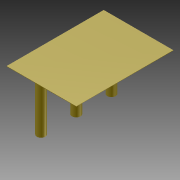
# Autodesk Inventor part: B12APtrmnls
Saved by Autodesk Inventor 2011 SP1 (Build 150282100, 282)
## iProperties
Created: 2013-12-24
Part Number: B12APtrmnls
Catalog Web Link: www.cadenas.de
Description: B Series - Terminals-
Vendor: NKKSWITCHES
Document SubType Name: Modeling
Designer: PARTuser1
Manufacturer: NKKSWITCHES
Density: 1 g/cm^3
Category: PARTsolutions
Company: NKKSWITCHES
Title: B12APtrmnls
Author: Cadenas PARTsolutions
PSOL_IDENT_0: {$CADENAS_DATA\23d-libs\nkkswitches\toggle\b\parts\b_terminals.prj},209 {VTYP=3D},{NB=B12APtrmnls},{
PSOL_IDENT_1: LINA=B12APtrmnls},{NN=B Series - Terminals},{DATE=06.03.2009 07:37:56},{GEOMDATE=28.01.2009 09:08:00
PSOL_IDENT_2: },{VERSION=},{LINEID=10},{LINESUBID=-1},{WBVAR=PLS,CRCTS,TGGLS,TRMNLS,CPS,CCLR}  {NB=B12APtrmnls},{L
PSOL_IDENT_3: INA=B12APtrmnls},{KT=DUMMY},{PN=B12AP},{SRS=B},{PLS=1},{CRCTS=2},{CRCTSALG= '2','2 - ON/NONE/ON','3'
PSOL_IDENT_4: ,'3 - ON/OFF/ON','5','5 - ON/NONE/(ON)','R','R - (ON)/NONE/ON','8','8 - (ON)/OFF/(ON)','9','9 - ON/O
PSOL_IDENT_5: FF/(ON)','S','S - (ON)/OFF/ON' },{TGGLS=A},{TGGLSALG=  'A','A - .394\" (10.0 mm) Bat','A1','A1 - .31
PSOL_IDENT_6: 5\" (8.0 mm) Bat with Panel Seal Threaded Bushing  '  ,'J','J - .248\" (6.3 mm) Bat','E','E - .394\"
PSOL_IDENT_7: (10.0 mm) Flatted','H','H - .248\" (6.3 mm) Flatted','K','K - Snap Top for Paddles','L','L - Lockin
PSOL_IDENT_8: g Lever' },{TRMNLS=P},{TRMNLSALG= 'P','P - Straight','B','B - Straight with Bracket', 'H','H - Right
PSOL_IDENT_9: Angle with Bracket','V','V - Vertical with Bracket' ,'W','W - Straight Long' },{CPS=},{CPSALG= '','
PSOL_IDENT_10: w/o Cap','G','G - .394\" (10.0 mm) Bat Lever Cap' },{CCLR=},{CCLR1= '', 'N/A' }
CNS_NN: B Series - Terminals
CNS_NB: B12APtrmnls
CNS_NBSYN: $PN.trmnls
CNS_LINA: B12APtrmnls
CNS_PN: B12AP
CNS_SRS: B
CNS_PLS: 1 - SPDT
CNS_CRCTS: 2 - ON/NONE/ON
CNS_CRCTSALG: '2','2 - ON/NONE/ON','3','3 - ON/OFF/ON','5','5 - ON/NONE/(ON)','R','R - (ON)/NONE/ON','8','8 - (ON)/OFF/(ON)','9','9 - ON/OFF/(ON)','S','S - (ON)/OFF/ON'
CNS_TGGLS: A - .394" (10.0 mm) Bat
CNS_TGGLSALG: 'A','A - .394" (10.0 mm) Bat','A1','A1 - .315" (8.0 mm) Bat with Panel Seal Threaded Bushing  '  ,'J','J - .248" (6.3 mm) Bat','E','E - .394" (10.0 mm) Flatted','H','H - .248" (6.3 mm) Flatted','K','K - Snap Top for Paddles','L','L - Locking Lever'
CNS_TRMNLS: P - Straight
CNS_TRMNLSALG: 'P','P - Straight','B','B - Straight with Bracket', 'H','H - Right Angle with Bracket','V','V - Vertical with Bracket' ,'W','W - Straight Long'
CNS_CPS: w/o Cap
CNS_CPSALG: '','w/o Cap','G','G - .394" (10.0 mm) Bat Lever Cap'
CNS_CCLR: N/A
CNS_CCLR1: '', 'N/A'
SUPPLIER: NKKSWITCHES
ARTICLENO: B12APtrmnls
BOMINFO: B12APtrmnls
CREATOR: CADENAS GmbH
Autodesk Inventor part; units mm, degrees
sketch "Sketch_1" plane through (0, 0, 0) normal (0, 1, 0) x (-1, 0, 0)
  line L0 (2.5146, 3.5052) -> (-2.5146, 3.5052)
  line L1 (-2.5146, 3.5052) -> (-2.5146, -3.5052)
  line L2 (-2.5146, -3.5052) -> (2.5146, -3.5052)
  line L3 (2.5146, -3.5052) -> (2.5146, 3.5052)
  constraints: 8 end point
extrude "Extrusion1" add sketch "Sketch_1" along normal blind 0.0254
sketch "Sketch_2" plane through (0, 0, 0) normal (0, 1, 0) x (-1, 0, 0)
  circle A0 centre (0.9906, 0) radius 0.3048
  constraints: 1 centre point
extrude "Extrusion2" add sketch "Sketch_2" against normal blind 3.9624
sketch "Sketch_3" plane through (0, 0, 0) normal (0, 1, 0) x (-1, 0, 0)
  circle A0 centre (0.9906, -2.54) radius 0.3048
  constraints: 1 centre point
extrude "Extrusion3" add sketch "Sketch_3" against normal blind 3.9624
sketch "Sketch_4" plane through (0, 0, 0) normal (0, 1, 0) x (-1, 0, 0)
  circle A0 centre (0.9906, 2.54) radius 0.3048
  constraints: 1 centre point
extrude "Extrusion4" add sketch "Sketch_4" against normal blind 3.9624
ref_plane "right_vertical_trmnls_XY" through (0, 0, 0) normal (0, 0, -1) x (1, 0, 0)
ref_plane "right_vertical_trmnls_YZ" through (0, 0, 0) normal (1, 0, 0) x (0, -1, 0)
ref_plane "right_vertical_trmnls_ZX" through (0, 0, 0) normal (0, -1, 0) x (0, 0, -1)
ref_plane "stright_trmnls_XY" through (0, 0, 0) normal (0, -1, 0) x (1, 0, 0)
ref_plane "stright_trmnls_YZ" through (0, 0, 0) normal (1, 0, 0) x (0, 0, 1)
ref_plane "stright_trmnls_ZX" through (0, 0, 0) normal (0, 0, 1) x (0, -1, 0)
body "Solid1"
